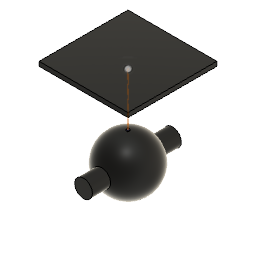
FPbasicmodel (Autodesk Fusion 360 design; units mm, degrees)
part number: 2025-10-07-19-33-31-705
Autodesk Fusion 360 part; units mm, degrees
sphere "SpherePrimitive1" add diameter 40 placed x (0, 1, 0) y (0, 0, 1) z (1, 0, 0) at (0, 0, 0) makes body 1
delete_face "DeleteFace1" 1 faces at (18.9615, 4.7276, -4.2557) on bodies 1
sphere "SpherePrimitive2" add diameter 250 placed x (0, 1, 0) y (0, 0, 1) z (1, 0, 0) at (0, 0, 0) separate body makes body 2
sketch "Sketch3" plane through (0, 0, 0) normal (1, 0, 0) x (0, 1, 0)
  line L0 (0, 0) -> (0, 125) construction
  line L1 (0, 125) -> (0, 375) construction
  line L2 (0, 375) -> (200, 375)
  line L3 (0, 375) -> (-200, 375)
  line L4 (-200, 375) -> (-200, 395)
  line L5 (-200, 395) -> (200, 395)
  line L6 (200, 395) -> (200, 375)
  dimension "d3" = 125
  dimension "d4" = 250
  dimension "d5" = 200
  dimension "d6" = 200
  dimension "d7" = 20
  constraint coincident L0.start origin
  constraint vertical L0
  constraint parallel L0 L1
  constraint perpendicular L1 L2
  constraint perpendicular L1 L3
  constraint perpendicular L3 L4
  constraint perpendicular L4 L5
  constraint perpendicular L2 L6
  measures "d3" distance of L0.start L0.end
  measures "d4" distance of L0.end L1.end
  measures "d5" distance of L1.end L2.end
  measures "d6" distance of L1.end L3.end
  measures "d7" distance of L3.end L4.end
extrude "Extrude1" add sketch "Sketch3" along normal blind 200 and the other way blind 200 separate body makes body 3
sketch "Sketch4" plane through (0, 0, 0) normal (0, 1, 0) x (1, 0, 0)
  circle A0 centre (0, 0) radius 40
  dimension "d12" = 80
  constraint coincident A0.centre origin
  measures "d12" diameter of A0
extrude "Extrude2" add sketch "Sketch4" along normal blind 200 and the other way blind 200 bodies 2
sketch "Sketch5" plane through (0, 0, 0) normal (0, 0, 1) x (1, 0, 0)
  line L0 (-5, 5) -> (5, 5)
  line L1 (5, 5) -> (5, -5)
  line L2 (5, -5) -> (-5, -5)
  line L3 (-5, -5) -> (-5, 5)
  line L4 (-5, 5) -> (5, -5) construction
  line L5 (5, 5) -> (-5, -5) construction
  dimension "d17" = 10
  dimension "d18" = 10
  constraint horizontal L0
  constraint perpendicular L0 L1
  constraint parallel L0 L2
  constraint parallel L1 L3
  constraint coincident L4 origin
  constraint coincident L5 origin
  measures "d17" distance of L1.end L2.end
  measures "d18" distance of L0.end L1.end
extrude "Extrude3" add sketch "Sketch5" along normal blind 10 from surface at 365 bodies 3
sketch "Sketch6" plane through (0, 0, 395) normal (0, 0, 1) x (-1, 0, 0)
  line L0 (200, 200) -> (-200, 200)
  line L1 (-200, 200) -> (-200, -200)
  line L2 (-200, -200) -> (200, -200)
  line L3 (200, -200) -> (200, 200)
  line L4 (-5, -5) -> (5, -5)
  line L5 (5, -5) -> (5, 5)
  line L6 (5, 5) -> (-5, 5)
  line L7 (-5, 5) -> (-5, -5)
  line L8 (-5, -5) -> (5, 5) construction
  line L9 (5, -5) -> (-5, 5) construction
  dimension "d22" = 10
  dimension "d23" = 10
  constraint horizontal L4
  constraint perpendicular L4 L5
  constraint parallel L4 L6
  constraint parallel L5 L7
  constraint coincident L8 origin
  constraint coincident L9 origin
  measures "d22" distance of L5.end L6.end
  measures "d23" distance of L4.end L5.end
extrude "Extrude4" add sketch "Sketch6" against normal blind 5 from surface at -265 contours L4 L5 L6 L7 bodies 2
sketch "Sketch7" plane through (0, 0, 0) normal (1, 0, 0) x (0, 1, 0)
  line L0 (-2.2071, 364.9003) -> (0, 130) construction
  line L1 (0, 130) -> (2.2298, 364.9003) construction
